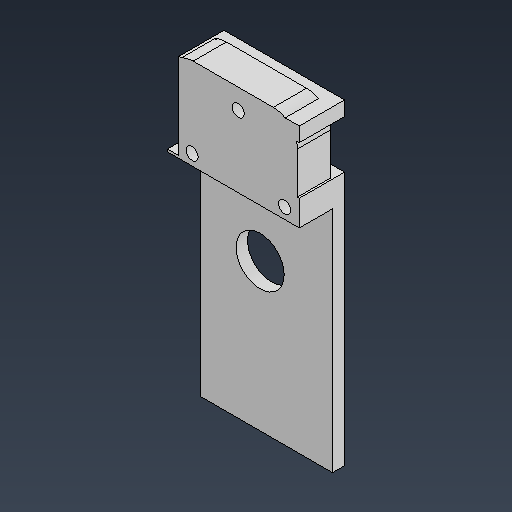
# Autodesk Inventor part: RightGearboxCover
Saved by Autodesk Inventor 2026.2 (Build 302298010, 298A)
## iProperties
Created: 2026-04-04
Part Number: RightGearboxCover
Material: Generic
Document SubType Name: Modeling
Designer: szymo
Density: 1 g/cm^3
Appearance: Default
Mass: 5.30599 g
Surface Area: 48.5829 cm^2
Volume: 5.30599 cm^3
Author: szymo
Autodesk Inventor part; units mm, degrees
ref_plane "YZ Plane" through (0, 0, 0) normal (1, 0, 0) x (0, 1, 0)
ref_plane "XZ Plane" through (0, 0, 0) normal (0, 1, 0) x (-1, 0, 0)
ref_plane "XY Plane" through (0, 0, 0) normal (0, 0, 1) x (1, 0, 0)
ref_plane "Work Plane1" through (0, -65.2958, -0.3) normal (0, 0, 1) x (1, 0, 0)
ref_plane "Work Plane4" through (0.0409, -65.2958, -0.1) normal (0, 0, 1) x (1, 0, 0)
sketch "Sketch1" plane through (0, 0, 0) normal (0, 0, 1) x (1, 0, 0)
  circle A0 centre (13, -35.9222) radius 5
  circle A1 centre (13, -35.9222) radius 5.6
  circle A2 centre (9.2216, -10.2077) radius 1.0564
  circle A3 centre (21.4784, -20.4923) radius 1.0564 construction
  circle A4 centre (15.35, -15.35) radius 5 construction
  circle A5 centre (15.35, -15.35) radius 14 construction
  circle A6 centre (15.35, -15.35) radius 14.7 construction
  circle A7 centre (15.35, -56.2871) radius 14.7 construction
  circle A8 centre (15.35, -56.2871) radius 14 construction
  line L0 (28.05, -0.65) -> (0.65, -0.65)
  line L1 (0.65, -0.65) -> (0.65, -66.4871)
  line L2 (0.65, -66.4871) -> (28.05, -66.4871)
  line L3 (28.05, -66.4871) -> (28.05, -0.65)
  line L4 (1, -17) -> (1, -13.9)
  line L5 (1, -13.9) -> (0, -13.9)
  line L6 (0, -13.9) -> (0, -18)
  line L7 (0, -18) -> (2.4477, -18)
  arc A9 (2.5, -17.9298) -> (2.4477, -18) centre (9.2084, -22.9852) ccw
  line L8 (2.5, -17.9298) -> (2.5, -17)
  line L9 (2.5, -17) -> (1, -17)
  line L10 (3, -0.65) -> (3, -18.5)
  line L11 (3, -18.5) -> (0.65, -18.5)
  line L12 (3, -3.65) -> (28.05, -3.65)
  line L13 (28.05, -13.65) -> (3, -13.65)
  line L14 (23.6, -0.65) -> (23.6, -40.1959)
  arc A10 (8.7222, -28.8679) -> (7.5995, -27.9853) centre (4.4774, -33.1126) ccw
  arc A11 (7.5995, -27.9853) -> (7.1915, -28.2788) centre (13, -35.9222) ccw
  arc A12 (7.1915, -28.2788) -> (7.6714, -29.6239) centre (13.0453, -26.9485) ccw
  arc A13 (7.6714, -29.6239) -> (7.3491, -29.9114) centre (13, -35.9222) ccw
  arc A14 (7.3491, -29.9114) -> (6.0673, -29.2816) centre (4.0795, -34.946) ccw
  arc A15 (6.0673, -29.2816) -> (5.7293, -29.6535) centre (13, -35.9222) ccw
  arc A16 (5.7293, -29.6535) -> (6.4783, -30.8695) centre (11.1785, -27.1352) ccw
  arc A17 (6.4783, -30.8695) -> (6.2228, -31.2177) centre (13, -35.9222) ccw
  arc A18 (6.2228, -31.2177) -> (4.8381, -30.8681) centre (4.0714, -36.822) ccw
  arc A19 (4.8381, -30.8681) -> (4.5848, -31.3022) centre (13, -35.9222) ccw
  arc A20 (4.5848, -31.3022) -> (5.5703, -32.3358) centre (9.3914, -27.7059) ccw
  arc A21 (5.5703, -32.3358) -> (5.3928, -32.7296) centre (13, -35.9222) ccw
  arc A22 (5.3928, -32.7296) -> (3.9657, -32.6755) centre (4.4536, -38.6587) ccw
  arc A23 (3.9657, -32.6755) -> (3.8081, -33.1528) centre (13, -35.9222) ccw
  arc A24 (3.8081, -33.1528) -> (4.987, -33.9589) centre (7.762, -28.6357) ccw
  arc A25 (4.987, -33.9589) -> (4.8952, -34.3809) centre (13, -35.9222) ccw
  arc A26 (4.8952, -34.3809) -> (3.4881, -34.6248) centre (5.2093, -40.3758) ccw
  arc A27 (3.4881, -34.6248) -> (3.4332, -35.1244) centre (13, -35.9222) ccw
  arc A28 (3.4332, -35.1244) -> (4.7539, -35.6678) centre (6.3615, -29.884) ccw
  arc A29 (4.7539, -35.6678) -> (4.7519, -36.0997) centre (13, -35.9222) ccw
  arc A30 (4.7519, -36.0997) -> (3.4262, -36.6308) centre (6.3055, -41.8982) ccw
  arc A31 (3.4262, -36.6308) -> (3.4764, -37.1309) centre (13, -35.9222) ccw
  arc A32 (3.4764, -37.1309) -> (4.8812, -37.3878) centre (5.2512, -31.3962) ccw
  arc A33 (4.8812, -37.3878) -> (4.9691, -37.8107) centre (13, -35.9222) ccw
  arc A34 (4.9691, -37.8107) -> (3.7827, -38.6058) centre (7.6943, -43.1595) ccw
  arc A35 (3.7827, -38.6058) -> (3.9358, -39.0845) centre (13, -35.9222) ccw
  arc A36 (3.9358, -39.0845) -> (5.3633, -39.0438) centre (4.4795, -33.1061) ccw
  arc A37 (5.3633, -39.0438) -> (5.5372, -39.4392) centre (13, -35.9222) ccw
  arc A38 (5.5372, -39.4392) -> (4.5421, -40.4635) centre (9.3149, -44.1045) ccw
  arc A39 (4.5421, -40.4635) -> (4.7913, -40.9) centre (13, -35.9222) ccw
  arc A40 (4.7913, -40.9) -> (6.1792, -40.5633) centre (4.0802, -34.9392) ccw
  arc A41 (6.1792, -40.5633) -> (6.4315, -40.9139) centre (13, -35.9222) ccw
  arc A42 (6.4315, -40.9139) -> (5.6711, -42.1228) centre (11.0966, -44.6918) ccw
  arc A43 (5.6711, -42.1228) -> (6.0057, -42.4979) centre (13, -35.9222) ccw
  arc A44 (6.0057, -42.4979) -> (7.2932, -41.88) centre (4.0707, -36.8152) ccw
  arc A45 (7.2932, -41.88) -> (7.6128, -42.1705) centre (13, -35.9222) ccw
  arc A46 (7.6128, -42.1705) -> (7.1204, -43.5111) centre (12.9615, -44.8959) ccw
  arc A47 (7.1204, -43.5111) -> (7.5257, -43.8084) centre (13, -35.9222) ccw
  arc A48 (7.5257, -43.8084) -> (8.6566, -42.9363) centre (4.4515, -38.6522) ccw
  arc A49 (8.6566, -42.9363) -> (9.0297, -43.154) centre (13, -35.9222) ccw
  arc A50 (9.0297, -43.154) -> (8.8267, -44.5677) centre (14.8281, -44.7078) ccw
  arc A51 (8.8267, -44.5677) -> (9.2849, -44.7742) centre (13, -35.9222) ccw
  arc A52 (9.2849, -44.7742) -> (10.2098, -43.6861) centre (5.2059, -40.3699) ccw
  arc A53 (10.2098, -43.6861) -> (10.62, -43.8215) centre (13, -35.9222) ccw
  arc A54 (10.62, -43.8215) -> (10.7154, -45.2464) centre (16.6148, -44.1358) ccw
  arc A55 (10.7154, -45.2464) -> (11.2065, -45.3532) centre (13, -35.9222) ccw
  arc A56 (11.2065, -45.3532) -> (11.885, -44.0965) centre (6.301, -41.8931) ccw
  arc A57 (11.885, -44.0965) -> (12.3144, -44.1437) centre (13, -35.9222) ccw
  arc A58 (12.3144, -44.1437) -> (12.7039, -45.5176) centre (18.2435, -43.2047) ccw
  arc A59 (12.7039, -45.5176) -> (13.2065, -45.52) centre (13, -35.9222) ccw
  arc A60 (13.2065, -45.52) -> (13.6089, -44.1497) centre (7.6888, -43.1555) ccw
  arc A61 (13.6089, -44.1497) -> (14.0387, -44.1066) centre (13, -35.9222) ccw
  arc A62 (14.0387, -44.1066) -> (14.7054, -45.3695) centre (19.643, -41.9554) ccw
  arc A63 (14.7054, -45.3695) -> (15.1975, -45.2673) centre (13, -35.9222) ccw
  arc A64 (15.1975, -45.2673) -> (15.3062, -43.8433) centre (9.3087, -44.1017) ccw
  arc A65 (15.3062, -43.8433) -> (15.7176, -43.7118) centre (13, -35.9222) ccw
  arc A66 (15.7176, -43.7118) -> (16.6323, -44.8085) centre (20.7522, -40.4424) ccw
  arc A67 (16.6323, -44.8085) -> (17.0924, -44.6062) centre (13, -35.9222) ccw
  arc A68 (17.0924, -44.6062) -> (16.9027, -43.1907) centre (11.09, -44.6904) ccw
  arc A69 (16.9027, -43.1907) -> (17.2778, -42.9765) centre (13, -35.9222) ccw
  arc A70 (17.2778, -42.9765) -> (18.4005, -43.8591) centre (21.5226, -38.7318) ccw
  arc A71 (18.4005, -43.8591) -> (18.8085, -43.5656) centre (13, -35.9222) ccw
  arc A72 (18.8085, -43.5656) -> (18.3286, -42.2205) centre (12.9547, -44.8959) ccw
  arc A73 (18.3286, -42.2205) -> (18.6509, -41.933) centre (13, -35.9222) ccw
  arc A74 (18.6509, -41.933) -> (19.9327, -42.5628) centre (21.9205, -36.8985) ccw
  arc A75 (19.9327, -42.5628) -> (20.2707, -42.1909) centre (13, -35.9222) ccw
  arc A76 (20.2707, -42.1909) -> (19.5217, -40.975) centre (14.8215, -44.7092) ccw
  arc A77 (19.5217, -40.975) -> (19.7772, -40.6267) centre (13, -35.9222) ccw
  arc A78 (19.7772, -40.6267) -> (21.1619, -40.9763) centre (21.9286, -35.0224) ccw
  arc A79 (21.1619, -40.9763) -> (21.4152, -40.5422) centre (13, -35.9222) ccw
  arc A80 (21.4152, -40.5422) -> (20.4297, -39.5086) centre (16.6086, -44.1385) ccw
  arc A81 (20.4297, -39.5086) -> (20.6072, -39.1149) centre (13, -35.9222) ccw
  arc A82 (20.6072, -39.1149) -> (22.0343, -39.1689) centre (21.5464, -33.1858) ccw
  arc A83 (22.0343, -39.1689) -> (22.1919, -38.6917) centre (13, -35.9222) ccw
  arc A84 (22.1919, -38.6917) -> (21.013, -37.8855) centre (18.238, -43.2087) ccw
  arc A85 (21.013, -37.8855) -> (21.1048, -37.4635) centre (13, -35.9222) ccw
  arc A86 (21.1048, -37.4635) -> (22.5119, -37.2196) centre (20.7907, -31.4687) ccw
  arc A87 (22.5119, -37.2196) -> (22.5668, -36.7201) centre (13, -35.9222) ccw
  arc A88 (22.5668, -36.7201) -> (21.2461, -36.1766) centre (19.6385, -41.9604) ccw
  arc A89 (21.2461, -36.1766) -> (21.2481, -35.7447) centre (13, -35.9222) ccw
  arc A90 (21.2481, -35.7447) -> (22.5738, -35.2137) centre (19.6945, -29.9462) ccw
  arc A91 (22.5738, -35.2137) -> (22.5236, -34.7136) centre (13, -35.9222) ccw
  arc A92 (22.5236, -34.7136) -> (21.1188, -34.4566) centre (20.7488, -40.4483) ccw
  arc A93 (21.1188, -34.4566) -> (21.0309, -34.0337) centre (13, -35.9222) ccw
  arc A94 (21.0309, -34.0337) -> (22.2173, -33.2386) centre (18.3057, -28.6849) ccw
  arc A95 (22.2173, -33.2386) -> (22.0642, -32.7599) centre (13, -35.9222) ccw
  arc A96 (22.0642, -32.7599) -> (20.6367, -32.8007) centre (21.5205, -38.7383) ccw
  arc A97 (20.6367, -32.8007) -> (20.4628, -32.4053) centre (13, -35.9222) ccw
  arc A98 (20.4628, -32.4053) -> (21.4579, -31.3809) centre (16.6851, -27.74) ccw
  arc A99 (21.4579, -31.3809) -> (21.2087, -30.9445) centre (13, -35.9222) ccw
  arc A100 (21.2087, -30.9445) -> (19.8208, -31.2811) centre (21.9198, -36.9052) ccw
  arc A101 (19.8208, -31.2811) -> (19.5685, -30.9305) centre (13, -35.9222) ccw
  arc A102 (19.5685, -30.9305) -> (20.3289, -29.7216) centre (14.9034, -27.1526) ccw
  arc A103 (20.3289, -29.7216) -> (19.9943, -29.3466) centre (13, -35.9222) ccw
  arc A104 (19.9943, -29.3466) -> (18.7068, -29.9644) centre (21.9293, -35.0292) ccw
  arc A105 (18.7068, -29.9644) -> (18.3872, -29.6739) centre (13, -35.9222) ccw
  arc A106 (18.3872, -29.6739) -> (18.8796, -28.3334) centre (13.0385, -26.9485) ccw
  arc A107 (18.8796, -28.3334) -> (18.4743, -28.0361) centre (13, -35.9222) ccw
  arc A108 (18.4743, -28.0361) -> (17.3434, -28.9081) centre (21.5485, -33.1922) ccw
  arc A109 (17.3434, -28.9081) -> (16.9703, -28.6904) centre (13, -35.9222) ccw
  arc A110 (16.9703, -28.6904) -> (17.1733, -27.2768) centre (11.1719, -27.1366) ccw
  arc A111 (17.1733, -27.2768) -> (16.7151, -27.0702) centre (13, -35.9222) ccw
  arc A112 (16.7151, -27.0702) -> (15.7902, -28.1584) centre (20.7941, -31.4746) ccw
  arc A113 (15.7902, -28.1584) -> (15.38, -28.023) centre (13, -35.9222) ccw
  arc A114 (15.38, -28.023) -> (15.2846, -26.598) centre (9.3852, -27.7087) ccw
  arc A115 (15.2846, -26.598) -> (14.7935, -26.4912) centre (13, -35.9222) ccw
  arc A116 (14.7935, -26.4912) -> (14.115, -27.7479) centre (19.699, -29.9513) ccw
  arc A117 (14.115, -27.7479) -> (13.6856, -27.7008) centre (13, -35.9222) ccw
  arc A118 (13.6856, -27.7008) -> (13.2961, -26.3268) centre (7.7565, -28.6397) ccw
  arc A119 (13.2961, -26.3268) -> (12.7935, -26.3244) centre (13, -35.9222) ccw
  arc A120 (12.7935, -26.3244) -> (12.3911, -27.6947) centre (18.3112, -28.689) ccw
  arc A121 (12.3911, -27.6947) -> (11.9613, -27.7379) centre (13, -35.9222) ccw
  arc A122 (11.9613, -27.7379) -> (11.2946, -26.4749) centre (6.357, -29.889) ccw
  arc A123 (11.2946, -26.4749) -> (10.8025, -26.5771) centre (13, -35.9222) ccw
  arc A124 (10.8025, -26.5771) -> (10.6938, -28.0011) centre (16.6913, -27.7428) ccw
  arc A125 (10.6938, -28.0011) -> (10.2824, -28.1327) centre (13, -35.9222) ccw
  arc A126 (10.2824, -28.1327) -> (9.3677, -27.0359) centre (5.2478, -31.4021) ccw
  arc A127 (9.3677, -27.0359) -> (8.9076, -27.2382) centre (13, -35.9222) ccw
  arc A128 (8.9076, -27.2382) -> (9.0973, -28.6537) centre (14.91, -27.154) ccw
  arc A129 (9.0973, -28.6537) -> (8.7222, -28.8679) centre (13, -35.9222) ccw
  circle A130 centre (13, -35.9222) radius 9.6 construction
  point P0 (0, 0)
  point P1 (23.6, -13.65)
  point P2 (23.6, -3.65)
extrude "Extrusion1" add sketch "Sketch1" against normal up to surface (0.1 mm away) contours A2 | L3 L12 L14 L0 | L14 L12 L10 L0 | L14 L13 L10 L12 | L3 L2 L1 L11 L10 L13 | A129 A128 A127 A126 A125 A124 A123 A122 A121 A120 A119 A118 A117 A116 A115 A114 A113 A112 A111 A110 A109 A108 A107 A106 A105 A104 A103 A102 A101 A100 A99 A98 A97 A96 A95 A94 A93 A92 A91 A90 A89 A88 A87 A86 A85 A84 A83 A82 A81 A80 A79 A78 A77 A76 A75 A74 A73 A72 A71 A70 A69 A68 A67 A66 A65 A64 A63 A62 A61 A60 A59 A58 A57 A56 A55 A54 A53 A52 A51 A50 A49 A48 A47 A46 A45 A44 A43 A42 A41 A40 A39 A38 A37 A36 A35 A34 A33 A32 A31 A30 A29 A28 A27 A26 A25 A24 A23 A22 A21 A20 A19 A18 A17 A16 A15 A14 A13 A12 A11 A10
ref_plane "Work Plane2" through (8.0794, -39.9218, 2.4) normal (0, 0, 1) x (0.9996763, -0.0254413, 0)
extrude "Extrusion2" add sketch "Sketch1" along normal up to surface (2.4 mm away) contours A1 | A2 | L3 L12 L14 L0 | L14 L12 L10 L0 | L14 L13 L10 L12 | L3 L2 L1 L11 L10 L13 | A129 A128 A127 A126 A125 A124 A123 A122 A121 A120 A119 A118 A117 A116 A115 A114 A113 A112 A111 A110 A109 A108 A107 A106 A105 A104 A103 A102 A101 A100 A99 A98 A97 A96 A95 A94 A93 A92 A91 A90 A89 A88 A87 A86 A85 A84 A83 A82 A81 A80 A79 A78 A77 A76 A75 A74 A73 A72 A71 A70 A69 A68 A67 A66 A65 A64 A63 A62 A61 A60 A59 A58 A57 A56 A55 A54 A53 A52 A51 A50 A49 A48 A47 A46 A45 A44 A43 A42 A41 A40 A39 A38 A37 A36 A35 A34 A33 A32 A31 A30 A29 A28 A27 A26 A25 A24 A23 A22 A21 A20 A19 A18 A17 A16 A15 A14 A13 A12 A11 A10
sketch "Sketch2" plane through (28.05, -66.4871, -0.1) normal (0, 0, -1) x (-1, 0, 0)
  circle A0 centre (12.5, 50.7958) radius 1.15 projected
  circle A1 centre (12.5, 50.7958) radius 1.65
  circle A2 centre (17.7916, 42.3106) radius 3 projected
  point P0 (28.05, 66.4871)
  dimension "d9" = 0.5
  constraints: 1 centre point
  measures "d9" radial gap between concentric circles of A0 A1
extrude "Extrusion3" cut sketch "Sketch2" against normal blind 2 contours A0 | A1
ref_plane "Work Plane3" through (1, -19, 8.2) normal (0, 0, -1) x (0, 1, 0)
ref_plane "Work Plane5" through (1, -19, 9.3) normal (0, 0, -1) x (0, 1, 0)
sketch "Sketch4" plane through (0.65, -66.4871, 2.4) normal (0, 0, 1) x (1, 0, 0)
  circle A0 centre (13.675, 63.4871) radius 0.75 projected
  circle A1 centre (4.075, 50.938) radius 0.75 projected
  circle A2 centre (23.275, 50.938) radius 0.75 projected
  line L0 (23.1168, 47.4871) -> (4.2332, 47.4871) projected
  arc A3 (4.2332, 47.4871) -> (4.1944, 47.4901) centre (4.175, 46.9905) ccw projected
  arc A4 (0.35, 51.4871) -> (4.1944, 47.4901) centre (4.35, 51.4871) ccw projected
  line L1 (0.35, 61.4871) -> (0.35, 51.4871) projected
  arc A5 (5.35, 66.4871) -> (0.35, 61.4871) centre (5.35, 61.4871) ccw projected
  line L2 (22, 66.4871) -> (5.35, 66.4871) projected
  arc A6 (27, 61.4871) -> (22, 66.4871) centre (22, 61.4871) ccw projected
  line L3 (27, 51.4871) -> (27, 61.4871) projected
  arc A7 (23.1556, 47.4901) -> (27, 51.4871) centre (23, 51.4871) ccw projected
  arc A8 (23.1556, 47.4901) -> (23.1168, 47.4871) centre (23.175, 46.9905) ccw projected
  line L4 (22.95, 52.8371) -> (2.35, 52.8371)
  line L5 (2.35, 47.9871) -> (2.35, 65.8371) projected
  line L6 (27.4, 52.8371) -> (27.4, 0) projected
  line L7 (27.4, 47.4871) -> (0, 47.4871)
  line L8 (0, 0) -> (0, 47.9871) projected
  line L9 (22.95, 61.7371) -> (2.35, 61.7371)
  line L10 (2.35, 65.8371) -> (27.4, 65.8371) projected
  line L11 (2.35, 65.8371) -> (27.4, 65.8371) projected
  line L12 (22.95, 52.8371) -> (27.4, 52.8371) projected
  line L13 (22.95, 52.8371) -> (27.4, 52.8371) projected
  line L14 (27.4, 65.8371) -> (27.4, 62.8371) projected
  line L15 (27.4, 62.8371) -> (22.95, 62.8371) projected
  line L16 (22.95, 62.8371) -> (22.95, 52.8371) projected
  line L17 (0, 47.9871) -> (2.35, 47.9871) projected
  line L18 (2.35, 47.9871) -> (0, 47.9871)
  point P0 (-0.65, 66.4871)
  point P1 (4.2332, 47.4871)
  point P2 (23.1168, 47.4871)
  point P3 (22.65, 65.2958)
  point P4 (6, 65.2958)
  point P5 (2.35, 48.023)
  point P6 (2.35, 65.4871)
  point P7 (24.4653, 65.8371)
  point P8 (2.8847, 65.8371)
  point P9 (27.4, 63.3295)
  point P10 (4.2332, 47.4871)
  point P11 (23.1168, 47.4871)
  point P12 (27.4, 50.1038)
  point P13 (26.8143, 62.8371)
  point P14 (1.8103, 48.1236)
  dimension "d15" = 1
  constraints: 8 end point, 5 point on line, 2 horizontal, 1 collinear, 1 parallel, 1 perpendicular
  measures "d15" distance edge to line of A0 L9
extrude "Extrusion4" add sketch "Sketch4" along normal up to surface (6.9 mm away) contours A0 | A1 | A2 | L0 A3 A4 L5 L4 L12 L3 A7 A8 | A8 A7 L3 L12 L6 L7 | L7 L8 L17 L5 A4 A3 | L12 L16 L15 A6 L3 | L5 L9 L16 L4 | L5 A5 L10 A6 L15 L16 L9 | A6 L10 L14 L15 | L5 L10 A5 | L10 A5 L2 A6
sketch "Sketch5" plane through (28.05, -66.4871, -0.1) normal (0, 0, -1) x (-1, 0, 0)
  circle A0 centre (12.675, 62.2958) radius 0.75 projected
  circle A1 centre (22.275, 49.7467) radius 0.75 projected
  circle A2 centre (3.075, 49.7467) radius 0.75 projected
  line L0 (3.2332, 46.2958) -> (22.1168, 46.2958) projected
  arc A3 (22.1556, 46.2989) -> (22.1168, 46.2958) centre (22.175, 45.7992) ccw projected
  arc A4 (22.1556, 46.2989) -> (26, 50.2958) centre (22, 50.2958) ccw projected
  line L1 (26, 60.2958) -> (26, 50.2958) projected
  arc A5 (26, 60.2958) -> (21, 65.2958) centre (21, 60.2958) ccw projected
  line L2 (4.35, 65.2958) -> (21, 65.2958) projected
  arc A6 (4.35, 65.2958) -> (-0.65, 60.2958) centre (4.35, 60.2958) ccw projected
  line L3 (-0.65, 50.2958) -> (-0.65, 60.2958) projected
  arc A7 (-0.65, 50.2958) -> (3.1944, 46.2989) centre (3.35, 50.2958) ccw projected
  arc A8 (3.2332, 46.2958) -> (3.1944, 46.2989) centre (3.175, 45.7992) ccw projected
  point P0 (28.05, 66.4871)
hole "Hole1" at (24.975, -16.7403, -0.1) at (15.375, -4.1912, -0.1) at (5.775, -16.7403, -0.1) direction (0, 0, 1) diameter 3 depth 4.5 counterbore diameter 3.5 counterbore depth 0.5
hole "Hole2" at (24.975, -16.7403, -0.1) at (15.375, -4.1912, -0.1) at (5.775, -16.7403, -0.1) direction (0, 0, 1) diameter 2.5 end through all
hole "Hole3" at (10.2584, -24.1765, -0.1) direction (0, 0, 1) diameter 2.5 depth 2
sketch "Sketch6" plane through (0.65, -66.4871, 2.4) normal (0, 0, 1) x (1, 0, 0)
  ellipse E0 centre (4.4967, -7.3489) end of major axis (2.7203, -5.968) minor radius 2.25 projected
  ellipse E1 centre (-16.2255, -7.7288) end of major axis (-17.8045, -6.5013) minor radius 2 projected
  ellipse E2 centre (29.1767, 25.2149) end of major axis (27.5977, 26.4423) minor radius 2 projected
  ellipse E3 centre (-7.241, 6.5413) end of major axis (-8.82, 7.7688) minor radius 2 (-9.1777, 7.0406) -> (-8.2026, 8.295) ccw projected
  ellipse E4 centre (18.1498, 12.1909) end of major axis (16.3734, 13.5718) minor radius 2.25 (15.9778, 11.6034) -> (18.4324, 14.4231) ccw projected
  ellipse E5 centre (-7.2411, 6.5412) end of major axis (-9.0175, 7.922) minor radius 2.25 (-9.4889, 6.6402) -> (-7.8915, 8.6951) ccw projected
  point P0 (-0.65, 66.4871)
  point P1 (19.7, 61.7958)
  constraints: 6 other
hole "Hole4" [suppressed]
body "Solid1"
